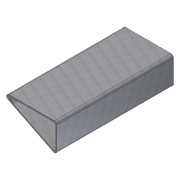
# Autodesk Inventor part: BatteryMount
Saved by Autodesk Inventor 2012 (Build 160160000, 160)
## iProperties
Created: 2012-02-23
Part Number: BatteryMount
Material: Aluminum-6061
Document SubType Name: Modeling
Designer: JesseK
Mass: 123.663 g
Surface Area: 509.027 cm^2
Volume: 45.6322 cm^3
Density: 2.71 g/cm^3
Author: JesseK
Autodesk Inventor part; units mm, degrees
ref_plane "YZ Plane" through (0, 0, 0) normal (1, 0, 0) x (0, 1, 0)
ref_plane "XZ Plane" through (0, 0, 0) normal (0, 1, 0) x (-1, 0, 0)
ref_plane "XY Plane" through (0, 0, 0) normal (0, 0, 1) x (1, 0, 0)
sketch "Sketch1" plane through (0, 0, 0) normal (0, 0, 1) x (1, 0, 0)
  line L0 (-3.175, 0) -> (-54.4382, 0)
  line L1 (-55.8581, -6.0148) -> (-4.5949, -31.6464)
  line L2 (0, -28.8066) -> (0, -3.175)
  line L3 (-1.5875, 1.5875) -> (-61.163, 1.5875)
  line L4 (-62.5829, -4.4273) -> (-3.0074, -34.215)
  line L5 (1.5875, -31.3752) -> (1.5875, -1.5875)
  arc A0 (-54.4382, 0) -> (-55.8581, -6.0148) centre (-54.4382, -3.175) ccw
  arc A1 (-61.163, 1.5875) -> (-62.5829, -4.4273) centre (-61.163, -1.5875) ccw
  arc A2 (-4.5949, -31.6464) -> (0, -28.8066) centre (-3.175, -28.8066) ccw
  arc A3 (-3.0074, -34.215) -> (1.5875, -31.3752) centre (-1.5875, -31.3752) ccw
  arc A4 (0, -3.175) -> (-3.175, 0) centre (-3.175, -3.175) ccw
  arc A5 (1.5875, -1.5875) -> (-1.5875, 1.5875) centre (-1.5875, -1.5875) ccw
  point P0 (0, 0)
  point P1 (-67.8877, 0)
  point P2 (0, -33.9439)
  point P3 (1.5875, 1.5875)
  point P4 (-74.6125, 1.5875)
  point P5 (1.5875, -36.5125)
  dimension "d0" = 1.5875
  dimension "d1" = 1.5875
  dimension "d2" = 1.5875
  dimension "d3" = 76.2
  dimension "d4" = 38.1
  dimension "d7" = 3.175
  dimension "d8" = 3.175
  constraints: 12 end point, 12 point on circle, 12 point on line, 12 tangent, 6 centre point, 4 equal radius, 2 parallel, 1 horizontal, 1 perpendicular, 1 vertical
  measures "d0" distance between parallel lines of L3 L0
  measures "d1" distance between parallel lines of L5 L2
  measures "d2" distance between parallel lines of L4 L1
  measures "d3" distance of point (1.587, 1.587) point (-74.613, 1.587)
  measures "d4" distance of point (1.588, -36.513) point (1.587, 1.587)
  measures "d7" radius of A0
  measures "d8" radius of A2
extrude "Extrusion1" add sketch "Sketch1" along normal blind 152.4
body "Solid1"
